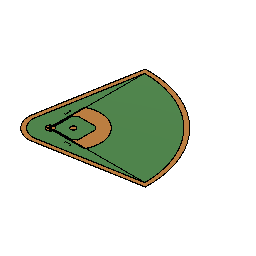
baseball_field_model (Autodesk Fusion 360 design; units mm, degrees)
Autodesk Fusion 360 part; units mm, degrees
sketch "Base Sketch" plane through (0, 0, 0) normal (0, 0, 1) x (1, 0, 0)
  line L0 (-60, -60) -> (340, -60)
  line L1 (340, -60) -> (340, 340)
  line L2 (340, 340) -> (-60, 340)
  line L3 (-60, 340) -> (-60, -60)
  circle A0 centre (0, 0) radius 60
  circle A1 centre (0, 0) radius 340
  line L4 (0, 0) -> (90, 0)
  line L5 (90, 0) -> (90, 90)
  line L6 (90, 90) -> (0, 90)
  line L7 (0, 90) -> (0, 0)
  circle A2 centre (0, 0) radius 13
  circle A3 centre (90, 0) radius 13
  circle A4 centre (90, 90) radius 13
  circle A5 centre (0, 90) radius 13
  line L8 (-3, 93) -> (-3, -3)
  line L9 (-3, -3) -> (93, -3)
  line L10 (93, -3) -> (93, 93)
  line L11 (93, 93) -> (-3, 93)
  line L12 (3, 87) -> (3, 3)
  line L13 (3, 3) -> (87, 3)
  line L14 (87, 3) -> (87, 87)
  line L15 (87, 87) -> (3, 87)
  line L16 (90, 90) -> (0, 0) construction
  circle A6 centre (41.7193, 41.7193) radius 9
  circle A7 centre (42.78, 42.78) radius 95
  line L17 (-3, 93) -> (-3, 126.0217)
  line L18 (93, -3) -> (126.0217, -3)
  line L19 (0, 0) -> (340, 0) construction
  line L20 (0, 0) -> (0, 340) construction
  point P0 (42.78, 42.78)
  point P1 (-3, 12.6491)
  point P2 (12.6491, -3)
  dimension "d3" = 400
  dimension "d4" = 400
  dimension "d5" = 120
  dimension "d6" = 90
  dimension "d7" = 90
  dimension "d8" = 26
  dimension "d9" = 26
  dimension "d10" = 26
  dimension "d11" = 26
  dimension "d12" = 3
  dimension "d13" = -3
  dimension "d14" = 18
  dimension "d15" = 59
  dimension "d16" = 1.5
  dimension "d17" = 190
  constraint horizontal L0
  constraint vertical L1
  constraint horizontal L2
  constraint vertical L3
  constraint tangent L0 A0
  constraint tangent L3 A0
  constraint concentric A0 A1
  constraint tangent L1 A1
  constraint horizontal L4
  constraint vertical L5
  constraint horizontal L6
  constraint vertical L7
  constraint coincident A0.centre A1.centre
  constraint concentric A0 A2
  constraint coincident L4.end L5.start
  constraint coincident L5.end L6.start
  constraint coincident L6.end L7.start
  constraint coincident L16 A6.centre
  constraint coincident L16 P0
  constraint coincident P0 A7.centre
  constraint perpendicular L11 L17
  constraint perpendicular L10 L18
  constraint coincident A2 P1
  constraint coincident L8 P1
  constraint coincident A2 P2
  constraint coincident L9 P2
  constraint coincident A1 L19.end
  constraint parallel L0 L19
  constraint coincident A1 L20.end
  constraint parallel L3 L20
  constraint coincident L0.start L3.end
  constraint coincident A7 L18.end
  constraint coincident A7 L17.end
  measures "d3" distance of L0.start L0.end
  measures "d4" distance of L0.start L2.end
  measures "d5" diameter of A0
  measures "d6" distance of A0.centre L4.end
  measures "d7" distance of A0.centre L6.end
  measures "d8" diameter of A2
  measures "d9" diameter of A3
  measures "d10" diameter of A4
  measures "d11" diameter of A5
  measures "d14" diameter of A6
  measures "d15" distance of A0.centre A6.centre
  measures "d16" distance of A6.centre P0
  measures "d17" diameter of A7
extrude "Extrude1" add sketch "Base Sketch" along normal blind 1 contours L0 L3 A0 A1 A7 | A0 A7 | A0 A2 L8 L9 A7 | A0 A3 L9 A7 L18 | A0 A5 L8 A7 L17 | A3 L9 L18 | A5 L8 L17 | A0 A2 L12 L13 A6 | A0 A3 A4 A5 L12 L13 L14 L15 A6 makes body 1 at (153.5619, -41, 0) makes body 2 at (74.8729, 44.3536, 0) in component "Grass"
sketch "Sketch1" plane through (0, 0, 1) normal (0, 0, 1) x (-1, 0, 0) in component "Grass"
  line L0 (3, -12.6491) -> (3, -126.0217)
  arc A0 (-126.0217, 3) -> (3, -126.0217) centre (-42.78, -42.78) ccw
  line L1 (-126.0217, 3) -> (-12.6491, 3)
  arc A1 (3, -12.6491) -> (-12.6491, 3) centre (0, 0) ccw
  arc A2 (-334.664, 60) -> (60, -334.664) centre (0, 0) ccw
  line L2 (60, -334.664) -> (60, 0)
  arc A3 (60, 0) -> (0, 60) centre (0, 0) ccw
  line L3 (0, 60) -> (-334.664, 60)
  line L4 (0, 0) -> (-340, 0)
  line L5 (0, 0) -> (0, -340)
  line L6 (0, 60) -> (-340, 0)
  line L7 (0, -340) -> (60, 0)
  constraint coincident A3.end L3.start
  constraint coincident L4.end L6.end
  constraint coincident L5.end L7.start
  constraint coincident L2.end A3.start
extrude "Extrude2" cut sketch "Sketch1" against normal up to surface (1 mm away) contours A2 L2 L7 | A2 L3 L6 bodies 1 in component "Grass"
sketch "Sketch1 (2)" plane through (0, 0, 0) normal (0, 0, 1) x (1, 0, 0) in component "Earth"
  line L0 (-60, -60) -> (340, -60)
  line L1 (340, -60) -> (340, 340)
  line L2 (340, 340) -> (-60, 340)
  line L3 (-60, 340) -> (-60, -60)
  line L4 (-75, 355) -> (-75, -75)
  line L5 (-75, -75) -> (355, -75)
  line L6 (355, -75) -> (355, 355)
  line L7 (355, 355) -> (-75, 355)
  dimension "d23" = 400
  dimension "d24" = 400
  dimension "d30" = 15
  dimension "d34" = 60
  dimension "d35" = 60
  constraint horizontal L0
  constraint vertical L1
  constraint horizontal L2
  constraint vertical L3
  measures "d23" distance of L0.start L0.end
  measures "d24" distance of L0.start L2.end
  measures "d34" distance of origin L3
  measures "d35" distance of origin L0
extrude "Extrude1'" add sketch "Sketch1 (2)" against normal blind 1 separate body contours L0 L1 L2 L3 | L4 L5 L6 L7 makes body 3 in component "Earth"
sketch "Sketch4" plane through (0, 0, 0) normal (0, 0, 1) x (1, 0, 0) in component "Dirt"
  line L0 (0, -60) -> (340, 0)
  arc A0 (340, 0) -> (0, 340) centre (0, 0) ccw
  line L1 (0, 340) -> (-60, 0)
  arc A1 (-60, 0) -> (0, -60) centre (0, 0) ccw
  line L2 (-3, 12.6491) -> (-3, 126.0217)
  arc A2 (126.0217, -3) -> (-3, 126.0217) centre (42.78, 42.78) ccw
  line L3 (126.0217, -3) -> (12.6491, -3)
  arc A3 (-3, 12.6491) -> (12.6491, -3) centre (0, 0) ccw
  circle A4 centre (41.7193, 41.7193) radius 9
  line L4 (3, 77.3509) -> (3, 12.6491)
  arc A5 (12.6491, 3) -> (3, 12.6491) centre (0, 0) ccw
  line L5 (12.6491, 3) -> (77.3509, 3)
  arc A6 (87, 12.6491) -> (77.3509, 3) centre (90, 0) ccw
  line L6 (87, 12.6491) -> (87, 77.3509)
  arc A7 (77.3509, 87) -> (87, 77.3509) centre (90, 90) ccw
  line L7 (77.3509, 87) -> (12.6491, 87)
  arc A8 (3, 77.3509) -> (12.6491, 87) centre (0, 90) ccw
  arc A9 (-74.9872, 1.386) -> (1.386, -74.9872) centre (0, 0) ccw
  line L8 (1.386, -74.9872) -> (354.7755, -12.6243)
  arc A10 (354.7755, -12.6243) -> (-12.6243, 354.7755) centre (0, 0) ccw
  line L9 (-12.6243, 354.7755) -> (-74.9872, 1.386)
  dimension "d31" = 15
extrude "Extrude1''" add sketch "Sketch4" along normal blind 1 separate body makes body 4 at (232.0538, -29.2038, 0) makes body 5 at (103.8497, 46.4661, 0) makes body 6 at (43.9778, 36.7996, 0) in component "Dirt"
ref_plane "WorkPlane1" through (0, 0, 1) normal (0, 0, 1) x (1, 0, 0) in component "Bases"
sketch "Sketch1 (3)" plane through (0, 0, 1) normal (0, 0, 1) x (1, 0, 0) in component "Bases"
  line L0 (77.3509, 3) -> (12.6491, 3)
  arc A0 (12.6491, 3) -> (3, 12.6491) centre (0, 0) ccw
  line L1 (3, 12.6491) -> (3, 77.3509)
  arc A1 (3, 77.3509) -> (12.6491, 87) centre (0, 90) ccw
  line L2 (12.6491, 87) -> (77.3509, 87)
  arc A2 (77.3509, 87) -> (87, 77.3509) centre (90, 90) ccw
  line L3 (87, 77.3509) -> (87, 12.6491)
  arc A3 (87, 12.6491) -> (77.3509, 3) centre (90, 0) ccw
  arc A4 (126.0217, -3) -> (-3, 126.0217) centre (42.78, 42.78) ccw
  line L4 (-3, 126.0217) -> (-3, 12.6491)
  arc A5 (-3, 12.6491) -> (12.6491, -3) centre (0, 0) ccw
  line L5 (12.6491, -3) -> (126.0217, -3)
  circle A6 centre (41.7193, 41.7193) radius 9
  line L6 (90, 0) -> (88.75, 0)
  line L7 (88.75, 0) -> (88.75, 1.25)
  line L8 (88.75, 1.25) -> (90, 1.25)
  line L9 (90, 1.25) -> (90, 0)
  line L10 (0, 90) -> (1.25, 90)
  line L11 (1.25, 90) -> (1.25, 88.75)
  line L12 (1.25, 88.75) -> (0, 88.75)
  line L13 (0, 88.75) -> (0, 90)
  line L14 (90.625, 89.375) -> (89.375, 89.375)
  line L15 (89.375, 89.375) -> (89.375, 90.625)
  line L16 (89.375, 90.625) -> (90.625, 90.625)
  line L17 (90.625, 90.625) -> (90.625, 89.375)
  line L18 (90.625, 89.375) -> (89.375, 90.625) construction
  line L19 (89.375, 89.375) -> (90.625, 90.625) construction
  line L20 (42.78, 42.78) -> (41.7193, 41.7193) construction
  line L21 (42.78, 42.78) -> (43.4871, 42.0729) construction
  line L22 (42.78, 42.78) -> (42.0729, 43.4871) construction
  line L23 (43.4871, 42.0729) -> (42.0729, 43.4871)
  line L24 (42.0729, 43.4871) -> (42.4264, 43.8406)
  line L25 (42.4264, 43.8406) -> (43.8406, 42.4264)
  line L26 (43.8406, 42.4264) -> (43.4871, 42.0729)
  line L27 (0, 0) -> (41.7193, 41.7193) construction
  line L28 (0, 0) -> (0, 1.0017)
  line L29 (0, 1.0017) -> (0.5009, 1.5026)
  line L30 (0.5009, 1.5026) -> (1.5026, 0.5009)
  line L31 (1.5026, 0.5009) -> (1.0017, 0)
  line L32 (0, 0) -> (1.0017, 0)
  point P0 (90, 90)
  dimension "d40" = 1.25
  dimension "d41" = 1.25
  dimension "d42" = 1.25
  dimension "d43" = 1.25
  dimension "d44" = 1.25
  dimension "d45" = 1.25
  dimension "d48" = 1
  dimension "d49" = 1
  dimension "d50" = 0.5
  dimension "d51" = 0.7083
  dimension "d52" = 1.4167
  constraint horizontal L6
  constraint vertical L7
  constraint horizontal L8
  constraint vertical L9
  constraint coincident A3.centre L6.start
  constraint horizontal L10
  constraint vertical L11
  constraint horizontal L12
  constraint vertical L13
  constraint coincident A1.centre L10.start
  constraint horizontal L14
  constraint perpendicular L14 L15
  constraint parallel L14 L16
  constraint parallel L15 L17
  constraint coincident L18 P0
  constraint coincident L19 P0
  constraint coincident P0 A2.centre
  constraint coincident A4.centre L20.start
  constraint coincident A6.centre L20.end
  constraint perpendicular L20 L21
  constraint perpendicular L20 L22
  constraint perpendicular L23 L24
  constraint parallel L23 L25
  constraint parallel L24 L26
  constraint coincident A0.centre A5.centre
  constraint vertical L28
  constraint parallel L27 L29
  constraint perpendicular L27 L30
  constraint perpendicular L30 L31
  constraint perpendicular L28 L32
  constraint coincident L31.end L32.end
  constraint equal L29 L31
  measures "d40" distance of A3.centre L6.end
  measures "d41" distance of A3.centre L8.end
  measures "d42" distance of A1.centre L10.end
  measures "d43" distance of A1.centre L12.end
  measures "d44" distance of L15.end L16.end
  measures "d45" distance of L14.end L15.end
  measures "d48" distance of A4.centre L21.end
  measures "d49" distance of A4.centre L22.end
  measures "d50" distance of L21.end L25.end
  measures "d51" distance of L28.end L29.end
  measures "d52" distance of L29.end L30.end
extrude "Extrude1'''" add sketch "Sketch1 (3)" along normal blind 0.25 separate body contours L6 L7 L8 L9 | L10 L11 L12 L13 | L14 L15 L16 L17 makes body 7 at (89.5833, 0.4167, 1) makes body 8 at (90.2083, 89.7917, 1) makes body 9 at (0.4167, 89.5833, 1) in component "Bases"
extrude "Extrude2'" add sketch "Sketch1 (3)" along normal blind 0.1 separate body contours L23 L24 L25 L26 | L28 L29 L30 L31 L32 makes body 10 at (0.3339, 0.3339, 1) makes body 11 at (43.2514, 42.78, 1) in component "Bases"
ref_plane "WorkPlane1" through (0, 0, 1) normal (0, 0, 1) x (1, 0, 0) in component "Lines"
sketch "Lines Sketch" plane through (0, 0, 1) normal (0, 0, 1) x (1, 0, 0) in component "Lines"
  circle A0 centre (41.7193, 41.7193) radius 9
  line L0 (3, 77.3509) -> (3, 12.6491)
  arc A1 (12.6491, 3) -> (3, 12.6491) centre (0, 0) ccw
  line L1 (12.6491, 3) -> (77.3509, 3)
  arc A2 (87, 12.6491) -> (77.3509, 3) centre (90, 0) ccw
  line L2 (87, 12.6491) -> (87, 77.3509)
  arc A3 (77.3509, 87) -> (87, 77.3509) centre (90, 90) ccw
  line L3 (77.3509, 87) -> (12.6491, 87)
  arc A4 (3, 77.3509) -> (12.6491, 87) centre (0, 90) ccw
  line L4 (0, 340) -> (-60, 0)
  arc A5 (-60, 0) -> (0, -60) centre (0, 0) ccw
  line L5 (0, -60) -> (340, 0)
  arc A6 (340, 0) -> (0, 340) centre (0, 0) ccw
  line L6 (-3, 12.6491) -> (-3, 126.0217)
  arc A7 (126.0217, -3) -> (-3, 126.0217) centre (42.78, 42.78) ccw
  line L7 (126.0217, -3) -> (12.6491, -3)
  arc A8 (-3, 12.6491) -> (12.6491, -3) centre (0, 0) ccw
  line L8 (0, 0) -> (41.7193, 41.7193) construction
  line L9 (-0.766, -2.4749) -> (3.4766, 1.7678)
  line L10 (3.4766, 1.7678) -> (6.305, -1.0607)
  line L11 (6.305, -1.0607) -> (2.0624, -5.3033)
  line L12 (2.0624, -5.3033) -> (-0.766, -2.4749)
  line L13 (-1.0607, 6.305) -> (1.7678, 3.4766)
  line L14 (-5.3033, 2.0624) -> (-1.0607, 6.305)
  line L15 (1.7678, 3.4766) -> (-2.4749, -0.766)
  line L16 (-2.4749, -0.766) -> (-5.3033, 2.0624)
  line L17 (-0.3536, -2.8874) -> (-4.39, -6.9238)
  line L18 (-4.39, -6.9238) -> (-6.9238, -4.39)
  line L19 (-6.9238, -4.39) -> (-2.8874, -0.3536)
  line L20 (0, 0) -> (340, 0) construction
  line L21 (0, 0) -> (0, 340) construction
  line L22 (5.2444, 0) -> (340, 0)
  line L23 (0, 5.2444) -> (0, 340)
  line L24 (5.2444, -0.2) -> (340, -0.2)
  line L25 (5.2444, 0.2) -> (340, 0.2)
  line L26 (-0.4832, -2.4749) -> (3.4766, 1.4849)
  line L27 (3.4766, 1.4849) -> (6.0222, -1.0607)
  line L28 (6.0222, -1.0607) -> (2.0624, -5.0205)
  line L29 (2.0624, -5.0205) -> (-0.4832, -2.4749)
  line L30 (-1.0489, -2.4749) -> (3.4766, 2.0506)
  line L31 (3.4766, 2.0506) -> (6.5879, -1.0607)
  line L32 (6.5879, -1.0607) -> (2.0624, -5.5861)
  line L33 (2.0624, -5.5861) -> (-1.0489, -2.4749)
  line L34 (0.2, 5.2444) -> (0.2, 340)
  line L35 (-0.2, 5.2444) -> (-0.2, 340)
  line L36 (-2.4749, -0.4832) -> (-5.0205, 2.0624)
  line L37 (-5.0205, 2.0624) -> (-1.0607, 6.0222)
  line L38 (-1.0607, 6.0222) -> (1.4849, 3.4766)
  line L39 (1.4849, 3.4766) -> (-2.4749, -0.4832)
  line L40 (-2.4749, -1.0489) -> (-5.5861, 2.0624)
  line L41 (-5.5861, 2.0624) -> (-1.0607, 6.5879)
  line L42 (-1.0607, 6.5879) -> (2.0506, 3.4766)
  line L43 (2.0506, 3.4766) -> (-2.4749, -1.0489)
  line L44 (-0.495, -2.7459) -> (-4.39, -6.6409)
  line L45 (-4.39, -6.6409) -> (-6.6409, -4.39)
  line L46 (-6.6409, -4.39) -> (-2.7459, -0.495)
  line L47 (-0.2121, -3.0288) -> (-4.39, -7.2066)
  line L48 (-4.39, -7.2066) -> (-7.2066, -4.39)
  line L49 (-7.2066, -4.39) -> (-3.0288, -0.2121)
  line L50 (340, -0.2) -> (340, 0.2)
  line L51 (0.2, 340) -> (-0.2, 340)
  line L52 (0, 90) -> (-20, 90) construction
  line L53 (-20, 90) -> (-15, 90)
  line L54 (-15, 90) -> (-15, 70)
  line L55 (-15, 70) -> (-20, 70)
  line L56 (-20, 89.8) -> (-15.2, 89.8)
  line L57 (-15.2, 89.8) -> (-15.2, 70.2)
  line L58 (-15.2, 70.2) -> (-20, 70.2)
  line L59 (-20, 90.2) -> (-14.8, 90.2)
  line L60 (-14.8, 90.2) -> (-14.8, 69.8)
  line L61 (-14.8, 69.8) -> (-20, 69.8)
  line L62 (-20, 90.2) -> (-20, 89.8)
  line L63 (-20, 70.2) -> (-20, 69.8)
  line L64 (90, 0) -> (90, -15) construction
  line L65 (90, -15) -> (90, -20)
  line L66 (90, -15) -> (70, -15)
  line L67 (70, -15) -> (70, -20)
  line L68 (69.8, -14.8) -> (69.8, -20)
  line L69 (90.2, -14.8) -> (69.8, -14.8)
  line L70 (90.2, -14.8) -> (90.2, -20)
  line L71 (70.2, -15.2) -> (70.2, -20)
  line L72 (89.8, -15.2) -> (70.2, -15.2)
  line L73 (89.8, -15.2) -> (89.8, -20)
  line L74 (90.2, -20) -> (89.8, -20)
  line L75 (70.2, -20) -> (69.8, -20)
  line L76 (0, 0) -> (-9.1924, -9.1924) construction
  line L77 (-9.1924, -9.1924) -> (16.9706, -35.3553) construction
  line L78 (-9.1924, -9.1924) -> (-35.3553, 16.9706) construction
  circle A9 centre (-35.3553, 16.9706) radius 2.5
  circle A10 centre (16.9706, -35.3553) radius 2.5
  circle A11 centre (16.9706, -35.3553) radius 2.7
  circle A12 centre (16.9706, -35.3553) radius 2.3
  circle A13 centre (-35.3553, 16.9706) radius 2.7
  circle A14 centre (-35.3553, 16.9706) radius 2.3
  line L79 (0, 88.75) -> (1.25, 88.75)
  line L80 (1.25, 88.75) -> (1.25, 90)
  line L81 (1.25, 90) -> (0, 90)
  line L82 (0, 90) -> (0, 88.75)
  line L83 (90, 1.25) -> (88.75, 1.25)
  line L84 (88.75, 1.25) -> (88.75, 0)
  line L85 (88.75, 0) -> (90, 0)
  line L86 (90, 0) -> (90, 1.25)
  line L87 (90.625, 90.625) -> (89.375, 90.625)
  line L88 (89.375, 90.625) -> (89.375, 89.375)
  line L89 (89.375, 89.375) -> (90.625, 89.375)
  line L90 (90.625, 89.375) -> (90.625, 90.625)
  dimension "d58" = 4
  dimension "d59" = 6
  dimension "d61" = 4
  dimension "d62" = 6
  dimension "d66" = 3.5833
  dimension "d67" = 8
  dimension "d69" = 0.2
  dimension "d70" = -0.2
  dimension "d71" = 0.2
  dimension "d72" = -0.2
  dimension "d73" = 0.2
  dimension "d74" = -0.2
  dimension "d75" = 0.2
  dimension "d76" = -0.2
  dimension "d77" = 0.2
  dimension "d78" = -0.2
  dimension "d84" = 5
  dimension "d85" = 20
  dimension "d86" = 5
  dimension "d87" = 0.2
  dimension "d88" = -0.2
  dimension "d89" = 15
  dimension "d90" = 15
  dimension "d91" = 5
  dimension "d92" = 20
  dimension "d93" = 5
  dimension "d94" = 0.2
  dimension "d95" = -0.2
  dimension "d96" = 37
  dimension "d97" = 37
  dimension "d98" = 5
  dimension "d99" = 5
  dimension "d100" = 0.2
  dimension "d101" = -0.2
  dimension "d102" = 0.2
  dimension "d103" = -0.2
  constraint coincident A1.centre A5.centre
  constraint coincident A0.centre L8.end
  constraint perpendicular L9 L10
  constraint parallel L9 L11
  constraint parallel L10 L12
  constraint perpendicular L13 L14
  constraint parallel L14 L15
  constraint parallel L13 L16
  constraint coincident L12 L17.start
  constraint perpendicular L12 L17
  constraint perpendicular L9 L18
  constraint coincident L16 L19.end
  constraint perpendicular L16 L19
  constraint symmetric L8 L17 L19
  constraint coincident L5.end A6.start
  constraint coincident L4.start A6.end
  constraint coincident L20 L22.start
  constraint coincident L10 L22.start
  constraint coincident L13 L23.start
  constraint coincident L21 L23.start
  constraint perpendicular L25 L50
  constraint perpendicular L34 L51
  constraint coincident A4.centre L52.start
  constraint perpendicular L6 L52
  constraint parallel L52 L53
  constraint perpendicular L52 L54
  constraint perpendicular L54 L55
  constraint perpendicular L56 L62
  constraint perpendicular L61 L63
  constraint coincident A2.centre L64.start
  constraint perpendicular L24 L64
  constraint parallel L64 L65
  constraint perpendicular L65 L66
  constraint perpendicular L66 L67
  constraint perpendicular L73 L74
  constraint perpendicular L68 L75
  constraint midpoint A8 L76.end
  constraint perpendicular L76 L77
  constraint perpendicular L76 L78
  constraint coincident L78.end A9.centre
  constraint coincident L77.end A10.centre
  measures "d58" distance of L9.start L11.end
  measures "d59" distance of L10.end L11.end
  measures "d61" distance of L14.start L15.end
  measures "d62" distance of L13.end L15.end
  measures "d66" distance of L17.end L18.end
  measures "d67" distance of A1.centre L18
  measures "d84" distance of L52.end L53.end
  measures "d85" distance of L53.end L54.end
  measures "d86" distance of L54.end L55.end
  measures "d89" distance of L21 L54
  measures "d90" distance of A2.centre L64.end
  measures "d91" distance of L64.end L65.end
  measures "d92" distance of L64.end L66.end
  measures "d93" distance of L66.end L67.end
  measures "d96" distance of L76.end L77.end
  measures "d97" distance of L76.end L78.end
  measures "d98" diameter of A9
  measures "d99" diameter of A10
extrude "Extrude1''''" add sketch "Lines Sketch" along normal blind 0.01 separate body contours L4 A7 L23 L35 | A6 A7 L23 L34 L51 | L4 L35 L51 | A7 L23 L35 L42 L82 | A7 L23 L34 L81 | A6 A7 L22 L25 L50 | L23 L34 L79 L81 L82 | L13 L23 L35 L42 | L13 L14 L16 L35 L40 L41 L42 L49 | L5 L24 L50 | L5 A7 L22 L24 | A7 L22 L25 L86 | L23 L34 L42 L79 | L13 L14 L15 L16 | L13 L15 L16 L23 L40 L42 L43 L46 | A7 L22 L24 L31 L85 | L22 L25 L84 L85 L86 | L22 L25 L31 L84 | L10 L11 L12 L24 L31 L32 L33 L47 | L10 L22 L24 L31 | L16 L19 L40 L49 | L17 L18 L19 L33 L40 L47 L48 L49 | L9 L10 L12 L22 L30 L31 L33 L44 | L9 L10 L11 L12 | L17 L18 L19 L33 L40 L44 L45 L46 | L16 L19 L40 L46 | L12 L17 L33 L47 | L12 L17 L33 L44 | L53 L54 L55 L59 L60 L61 L62 L63 | L53 L54 L55 L56 L57 L58 L62 L63 | L65 L66 L67 L68 L69 L70 L74 L75 | L65 L66 L67 L71 L72 L73 L74 L75 | A9 | A10 | A11 | A13 makes body 12 at (117.0181, 0.0667, 1) makes body 13 at (76.7333, -14.9333, 1) makes body 14 at (-14.9333, 76.7333, 1) makes body 15 at (-32.8073, 16.7222, 1) makes body 16 at (19.5186, -35.6037, 1) in component "Lines"
ref_plane "WorkPlane2" through (0, 0, 2.26) normal (0, 0, 1) x (1, 0, 0)
sketch "Final Sketch" plane through (0, 0, 2.26) normal (0, 0, 1) x (1, 0, 0)
  line L0 (-1.0607, 6.0222) -> (1.4849, 3.4766)
  line L1 (1.4849, 3.4766) -> (-2.4749, -0.4832)
  line L2 (-2.4749, -0.4832) -> (-5.0205, 2.0624)
  line L3 (-5.0205, 2.0624) -> (-1.0607, 6.0222)
  line L4 (6.0222, -1.0607) -> (2.0624, -5.0205)
  line L5 (2.0624, -5.0205) -> (-0.4832, -2.4749)
  line L6 (-0.4832, -2.4749) -> (3.4766, 1.4849)
  line L7 (3.4766, 1.4849) -> (6.0222, -1.0607)
  line L8 (0.2, 5.3272) -> (0.2, 339.9999)
  arc A0 (0.2, 339.9999) -> (0, 340) centre (0, 0) ccw
  line L9 (0, 340) -> (-0.2, 340)
  line L10 (-0.2, 340) -> (-0.2, 5.7272)
  line L11 (-0.2, 5.7272) -> (-1.0607, 6.5879)
  line L12 (-1.0607, 6.5879) -> (-5.5861, 2.0624)
  line L13 (-5.5861, 2.0624) -> (-3.1702, -0.3536)
  line L14 (-3.1702, -0.3536) -> (-7.2066, -4.39)
  line L15 (-7.2066, -4.39) -> (-4.39, -7.2066)
  line L16 (-4.39, -7.2066) -> (-0.3536, -3.1702)
  line L17 (-0.3536, -3.1702) -> (2.0624, -5.5861)
  line L18 (2.0624, -5.5861) -> (6.5879, -1.0607)
  line L19 (6.5879, -1.0607) -> (5.7272, -0.2)
  line L20 (5.7272, -0.2) -> (340, -0.2)
  line L21 (340, -0.2) -> (340, 0)
  arc A1 (340, 0) -> (339.9999, 0.2) centre (0, 0) ccw
  line L22 (339.9999, 0.2) -> (5.3272, 0.2)
  line L23 (5.3272, 0.2) -> (3.4766, 2.0506)
  line L24 (3.4766, 2.0506) -> (-1.0489, -2.4749)
  line L25 (-1.0489, -2.4749) -> (-0.6364, -2.8874)
  line L26 (-0.6364, -2.8874) -> (-4.39, -6.6409)
  line L27 (-4.39, -6.6409) -> (-6.6409, -4.39)
  line L28 (-6.6409, -4.39) -> (-2.8874, -0.6364)
  line L29 (-2.8874, -0.6364) -> (-2.4749, -1.0489)
  line L30 (-2.4749, -1.0489) -> (2.0506, 3.4766)
  line L31 (2.0506, 3.4766) -> (0.2, 5.3272)
  line L32 (0, 340) -> (-60, 0)
  arc A2 (-60, 0) -> (0, -60) centre (0, 0) ccw
  line L33 (0, -60) -> (340, 0)
  arc A3 (340, 0) -> (0, 340) centre (0, 0) ccw
  line L34 (-3, 12.6491) -> (-3, 126.0217)
  arc A4 (126.0217, -3) -> (-3, 126.0217) centre (42.78, 42.78) ccw
  line L35 (126.0217, -3) -> (12.6491, -3)
  arc A5 (-3, 12.6491) -> (12.6491, -3) centre (0, 0) ccw
  circle A6 centre (41.7193, 41.7193) radius 9
  line L36 (3, 77.3509) -> (3, 12.6491)
  arc A7 (12.6491, 3) -> (3, 12.6491) centre (0, 0) ccw
  line L37 (12.6491, 3) -> (77.3509, 3)
  arc A8 (87, 12.6491) -> (77.3509, 3) centre (90, 0) ccw
  line L38 (87, 12.6491) -> (87, 77.3509)
  arc A9 (77.3509, 87) -> (87, 77.3509) centre (90, 90) ccw
  line L39 (77.3509, 87) -> (12.6491, 87)
  arc A10 (3, 77.3509) -> (12.6491, 87) centre (0, 90) ccw
  line L40 (90, 1.25) -> (88.75, 1.25)
  line L41 (88.75, 1.25) -> (88.75, 0)
  line L42 (88.75, 0) -> (90, 0)
  line L43 (90, 0) -> (90, 1.25)
  line L44 (90.625, 90.625) -> (89.375, 90.625)
  line L45 (89.375, 90.625) -> (89.375, 89.375)
  line L46 (89.375, 89.375) -> (90.625, 89.375)
  line L47 (90.625, 89.375) -> (90.625, 90.625)
  line L48 (0, 88.75) -> (1.25, 88.75)
  line L49 (1.25, 88.75) -> (1.25, 90)
  line L50 (1.25, 90) -> (0, 90)
  line L51 (0, 90) -> (0, 88.75)
  line L52 (355, 355) -> (-75, 355)
  line L53 (-75, 355) -> (-75, -75)
  line L54 (-75, -75) -> (355, -75)
  line L55 (355, -75) -> (355, 355)
  arc A11 (-60, 0) -> (0, -60) centre (0, 0) ccw
  line L56 (-60, 0) -> (0, 340)
  arc A12 (340, 0) -> (0, 340) centre (0, 0) ccw
  line L57 (340, 0) -> (0, -60)
  line L58 (-12.6243, 354.7755) -> (-74.9872, 1.386)
  arc A13 (-74.9872, 1.386) -> (1.386, -74.9872) centre (0, 0) ccw
  line L59 (1.386, -74.9872) -> (354.7755, -12.6243)
  arc A14 (354.7755, -12.6243) -> (-12.6243, 354.7755) centre (0, 0) ccw
  circle A15 centre (-35.3553, 16.9706) radius 2.3
  circle A16 centre (-35.3553, 16.9706) radius 2.7
  line L60 (-20, 90.2) -> (-20, 89.8)
  line L61 (-20, 89.8) -> (-15.2, 89.8)
  line L62 (-15.2, 89.8) -> (-15.2, 70.2)
  line L63 (-15.2, 70.2) -> (-20, 70.2)
  line L64 (-20, 70.2) -> (-20, 69.8)
  line L65 (-20, 69.8) -> (-14.8, 69.8)
  line L66 (-14.8, 69.8) -> (-14.8, 90.2)
  line L67 (-14.8, 90.2) -> (-20, 90.2)
  line L68 (89.8, -15.2) -> (89.8, -20)
  line L69 (89.8, -20) -> (90.2, -20)
  line L70 (90.2, -20) -> (90.2, -14.8)
  line L71 (90.2, -14.8) -> (69.8, -14.8)
  line L72 (69.8, -14.8) -> (69.8, -20)
  line L73 (69.8, -20) -> (70.2, -20)
  line L74 (70.2, -20) -> (70.2, -15.2)
  line L75 (70.2, -15.2) -> (89.8, -15.2)
  circle A17 centre (16.9706, -35.3553) radius 2.3
  circle A18 centre (16.9706, -35.3553) radius 2.7
  line L76 (0, 88.75) -> (1.25, 88.75)
  line L77 (1.25, 88.75) -> (1.25, 90)
  line L78 (1.25, 90) -> (0, 90)
  line L79 (0, 90) -> (0, 88.75)
  line L80 (90, 1.25) -> (88.75, 1.25)
  line L81 (88.75, 1.25) -> (88.75, 0)
  line L82 (88.75, 0) -> (90, 0)
  line L83 (90, 0) -> (90, 1.25)
  line L84 (90.625, 90.625) -> (89.375, 90.625)
  line L85 (89.375, 90.625) -> (89.375, 89.375)
  line L86 (89.375, 89.375) -> (90.625, 89.375)
  line L87 (90.625, 89.375) -> (90.625, 90.625)
  line L88 (0, 88.75) -> (1.25, 88.75)
  line L89 (1.25, 88.75) -> (1.25, 90)
  line L90 (1.25, 90) -> (0, 90)
  line L91 (0, 90) -> (0, 88.75)
  line L92 (90, 1.25) -> (88.75, 1.25)
  line L93 (88.75, 1.25) -> (88.75, 0)
  line L94 (88.75, 0) -> (90, 0)
  line L95 (90, 0) -> (90, 1.25)
  line L96 (90.625, 90.625) -> (89.375, 90.625)
  line L97 (89.375, 90.625) -> (89.375, 89.375)
  line L98 (89.375, 89.375) -> (90.625, 89.375)
  line L99 (90.625, 89.375) -> (90.625, 90.625)
component "Grass" placed x (1, 0, 0) y (0, 1, 0) z (0, 0, 1) at (0, 0, 0)
component "Earth" placed x (1, 0, 0) y (0, 1, 0) z (0, 0, 1) at (0, 0, 0)
component "Dirt" placed x (1, 0, 0) y (0, 1, 0) z (0, 0, 1) at (0, 0, 0)
component "Bases" placed x (1, 0, 0) y (0, 1, 0) z (0, 0, 1) at (0, 0, 0)
component "Lines" placed x (1, 0, 0) y (0, 1, 0) z (0, 0, 1) at (0, 0, 0)
equation "d3 = Radius + 60 mm"
equation "d4 = Radius + 60 mm"
equation "d21 = Height"
equation "d23 = Radius + 60 mm"
equation "d24 = Radius + 60 mm"
equation "d25 = -Height"
equation "d30 = Padding"
equation "d31 = Padding"
equation "d32 = Height"
equation "Height = 1 mm"
equation "Padding = 15 mm"
equation "Radius = 340 mm"
equation "d39 = Height"
equation "d51 = ( 8.5 / 12 ) * 1 mm"
equation "d52 = ( 17 / 12 ) * 1 mm"
equation "d53 = BaseHeight"
equation "BaseHeight = 0.25 mm"
equation "d56 = Height"
equation "d66 = ( 43 / 12 ) * 1 mm"
equation "LineThickness = 0.4 mm"
equation "d69 = LineThickness / 2"
equation "d70 = -LineThickness / 2"
equation "d71 = LineThickness / 2"
equation "d72 = -LineThickness / 2"
equation "d73 = LineThickness / 2"
equation "d74 = -LineThickness / 2"
equation "d75 = LineThickness / 2"
equation "d76 = -LineThickness / 2"
equation "d77 = LineThickness / 2"
equation "d78 = -LineThickness / 2"
equation "d79 = LineHeight"
equation "LineHeight = 0.01 mm"
equation "d82 = 2 * Height + BaseHeight + LineHeight"
equation "d87 = LineThickness / 2"
equation "d88 = -LineThickness / 2"
equation "d94 = LineThickness / 2"
equation "d95 = -LineThickness / 2"
equation "d100 = LineThickness / 2"
equation "d101 = -LineThickness / 2"
equation "d102 = LineThickness / 2"
equation "d103 = -LineThickness / 2"
equation "HomePlateHeight = 0.1 mm"
equation "d105 = HomePlateHeight"
named bodies: "Outer Grass", "Inner Grass", "Earth", "Outer Dirt", "Main Dirt", "Pitcher Dirt", "First Base", "Second Base", "Third Base", "Lines", "Coach's Box 1", "Coach's Box 2", "Next Batter's Box 2", "Next Batter's Box 1", "Home Plate", "Pitcher's Mound"
